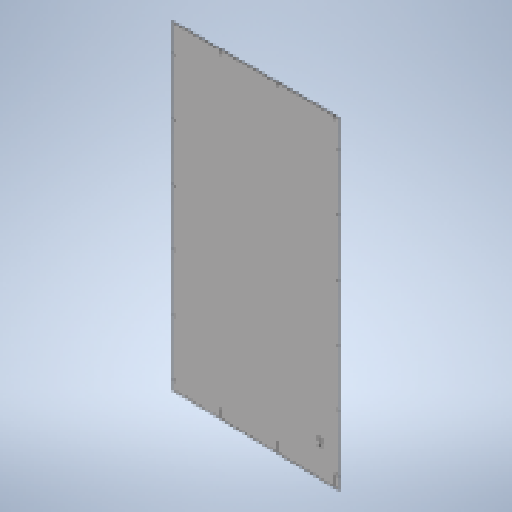
# Autodesk Inventor part: GBK 2211 shield 4
Saved by Autodesk Inventor 2026 (Build 300175000, 175)
## iProperties
Created: 2026-04-17
Part Number: GBK 2211 shield 4
Material: Steel
Document SubType Name: Sheet Metal
Designer: pokla
Stock Number: 2214
Mass: 138487 g
Surface Area: 88564.8 cm^2
Volume: 17641.6 cm^3
Density: 7.85 g/cm^3
Flat Pattern Width: 148 cm
Flat Pattern Length: 283.8 cm
Flat Pattern Area: 42002.4 cm^2
Sheet Metal Rule: По умолчанию_мм
Sheet Metal Width: 1480,000 мм
Sheet Metal Length: 2838,000 мм
Sheet Metal Area: 4200240,000 мм^2
Appearance: Default
Author: admin
Autodesk Inventor part; units mm, degrees
ref_plane "YZ Plane" through (0, 0, 0) normal (1, 0, 0) x (0, 1, 0)
ref_plane "XZ Plane" through (0, 0, 0) normal (0, 1, 0) x (-1, 0, 0)
ref_plane "XY Plane" through (0, 0, 0) normal (0, 0, 1) x (1, 0, 0)
sketch "Sketch1" plane through (0, 0, 0) normal (0, 0, 1) x (1, 0, 0)
  line L0 (740, -1490) -> (-740, -1490)
  line L1 (-740, -1490) -> (-740, 1490)
  line L2 (-740, 1490) -> (740, 1490)
  line L3 (740, 1490) -> (740, -1490)
  line L4 (740, -1490) -> (-740, 1490) construction
  line L5 (-740, -1490) -> (740, 1490) construction
  line L6 (740, -1348) -> (-740, -1314.4141)
  point P0 (0, 0)
  dimension "d0" = 1480
  dimension "d1" = 2980
  dimension "d3" = 1.3
  dimension "d5" = 2838
  dimension "d6" = 142
  measures "d0" distance of L1.end L2.end
  measures "d1" distance of L0.end L1.end
  measures "d3" angle of L0 L6
  measures "d5" distance of L6.start L2.end
  measures "d6" distance of L0.start L6.start
extrude "Plate1" add sketch "Sketch1" along normal blind 4 contours L6 L1 L2 L3
sketch "Sketch2" plane through (0, 0, 4) normal (0, 0, 1) x (1, 0, 0)
  line L0 (581.0754, -1023.615) -> (581.0754, -1381.3055) construction
  line L1 (581.0754, -1381.3055) -> (489.8191, -1381.3055) construction
  line L2 (489.8191, -1381.3055) -> (489.8191, -1023.615) construction
  line L3 (489.8191, -1023.615) -> (581.0754, -1023.615) construction
  line L4 (690.2486, -1244) -> (690.2486, -1341) projected
  line L5 (690.2486, -1341) -> (686.2496, -1341) projected
  line L6 (190.12, -1244) -> (190.12, -1341) projected
  line L7 (-310.0086, -1244) -> (-310.0086, -1341) projected
  line L8 (-310.0086, -1341) -> (-314.0076, -1341) projected
  line L9 (190.12, -1341) -> (186.121, -1341) projected
  ellipse E0 centre (-310.0086, 1484.5) end of major axis (-310.0086, 1514.5) minor radius 0.6803 (-310.0086, 1454.5) -> (-310.0086, 1514.5) ccw projected
  line L10 (-310.0086, 1454.5) -> (-314.0076, 1454.5) projected
  ellipse E1 centre (190.12, 1484.5) end of major axis (190.12, 1514.5) minor radius 0.6803 (190.12, 1454.5) -> (190.12, 1514.5) ccw projected
  line L11 (190.12, 1454.5) -> (186.121, 1454.5) projected
  ellipse E2 centre (690.2486, 1484.5) end of major axis (690.2486, 1514.5) minor radius 0.6803 (690.2486, 1454.5) -> (690.2486, 1514.5) ccw projected
  line L12 (690.2486, 1454.5) -> (686.2496, 1454.5) projected
  line L13 (770, 1246.8333) -> (710, 1246.8333) projected
  line L14 (710, 1242.8333) -> (710, 1246.8333) projected
  line L15 (770, 750.1667) -> (710, 750.1667) projected
  line L16 (710, 746.1667) -> (710, 750.1667) projected
  line L17 (770, 253.5) -> (710, 253.5) projected
  line L18 (710, 249.5) -> (710, 253.5) projected
  line L19 (770, -243.1667) -> (710, -243.1667) projected
  line L20 (710, -247.1667) -> (710, -243.1667) projected
  line L21 (770, -739.8333) -> (710, -739.8333) projected
  line L22 (710, -743.8333) -> (710, -739.8333) projected
  line L23 (770, -1236.5) -> (710, -1236.5) projected
  line L24 (710, -1240.5) -> (710, -1236.5) projected
  line L25 (-710, 1246.8333) -> (-739.3197, 1246.8333) projected
  line L26 (-710, 1242.8333) -> (-710, 1246.8333) projected
  line L27 (-710, 750.1667) -> (-739.3197, 750.1667) projected
  line L28 (-710, 746.1667) -> (-710, 750.1667) projected
  line L29 (-710, 253.5) -> (-739.3197, 253.5) projected
  line L30 (-710, 249.5) -> (-710, 253.5) projected
  line L31 (-710, -243.1667) -> (-739.3197, -243.1667) projected
  line L32 (-710, -247.1667) -> (-710, -243.1667) projected
  line L33 (-710, -739.8333) -> (-739.3197, -739.8333) projected
  line L34 (-710, -743.8333) -> (-710, -739.8333) projected
  line L35 (-710, -1236.5) -> (-739.3197, -1236.5) projected
  line L36 (-710, -1240.5) -> (-710, -1236.5) projected
  constraints: 5 other
mark "Mark1"
equation "\"d0\" = Лист_ширина"
equation "\"d2\" = Thickness"
equation "\"BendRadius\" = Thickness"
equation "\"BendReliefWidth\" = Thickness"
equation "\"BendReliefDepth\" = 0.5 * Thickness"
equation "\"CornerReliefSize\" = 4 * Thickness"
equation "\"MinimumRemnant\" = 2 * Thickness"
equation "\"TransitionRadius\" = BendRadius"
equation "\"JacobiRadiusSize\" = BendRadius"
equation "\"GapSize\" = Thickness"
equation "\"Лист_ширина\" = 1480"
equation "\"Thickness\" = 4"
body "Solid1"
